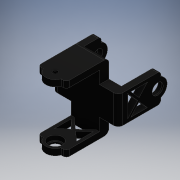
# Autodesk Inventor part: ServoArm
Saved by Autodesk Inventor 2016 (Build 200138000, 138)
## iProperties
Created: 2016-06-29
Part Number: ServoArm
Material: 一般
Document SubType Name: Modeling
Designer: Daisuke
Density: 1 g/cm^3
Appearance: 光沢 - 黒
Author: Daisuke
Autodesk Inventor part; units mm, degrees
ref_plane "YZ Plane" through (0, 0, 0) normal (1, 0, 0) x (0, 1, 0)
ref_plane "XZ Plane" through (0, 0, 0) normal (0, 1, 0) x (-1, 0, 0)
ref_plane "XY Plane" through (0, 0, 0) normal (0, 0, 1) x (1, 0, 0)
sketch "スケッチ1" plane through (0, 0, 0) normal (0, 1, 0) x (-1, 0, 0)
  line L0 (9, 20.9) -> (-9, 20.9)
  line L1 (-9, -20.9) -> (9, -20.9)
  line L2 (9, 20.9) -> (-9, -20.9) construction
  line L3 (-9, 20.9) -> (9, -20.9) construction
  line L4 (-20.9, 9) -> (-20.9, -9)
  line L5 (20.9, -9) -> (20.9, 9)
  line L6 (20.9, 9) -> (-20.9, -9) construction
  line L7 (-20.9, 9) -> (20.9, -9) construction
  line L8 (20.9, 9) -> (9, 9)
  line L9 (-9, 9) -> (-20.9, 9)
  line L10 (9, 9) -> (9, 20.9)
  line L11 (-9, 20.9) -> (-9, 9)
  line L12 (-9, -9) -> (-9, -20.9)
  line L13 (-20.9, -9) -> (-9, -9)
  line L14 (9, -9) -> (20.9, -9)
  line L15 (9, -20.9) -> (9, -9)
  point P0 (0, 0)
  dimension "d0" = 18
  dimension "d1" = 41.8
  dimension "d2" = 41.8
  dimension "d3" = 18
  constraints: 32 end point, 10 parallel, 4 midpoint, 4 perpendicular, 3 horizontal
  measures "d0" distance of L1.end L1.start
  measures "d1" distance of L1.start L0.end
  measures "d2" distance of L5.start L4.end
  measures "d3" distance of L4.end L4.start
extrude "押し出し1" add sketch "スケッチ1" along normal blind 6
sketch "スケッチ2" plane through (0, 6, 0) normal (0, 1, 0) x (1, 0, 0)
  line L0 (-20.9, -9) -> (-9, -9) projected
  line L1 (-9, 9) -> (-20.9, 9) projected
  line L2 (-20.9, -9) -> (-16.9, -9)
  line L3 (-16.9, -9) -> (-16.9, 9)
  line L4 (-16.9, 9) -> (-20.9, 9)
  line L5 (-20.9, 9) -> (-20.9, -9)
  line L6 (20.9, -9) -> (20.9, 9) projected
  line L7 (20.9, 9) -> (9, 9) projected
  line L8 (20.9, -9) -> (16.9, -9)
  line L9 (16.9, -9) -> (16.9, 9)
  line L10 (16.9, 9) -> (20.9, 9)
  line L11 (20.9, 9) -> (20.9, -9)
  point P0 (0, 0)
  dimension "d6" = 4
  dimension "d7" = 4
  constraints: 16 end point, 4 parallel, 2 horizontal, 2 perpendicular, 2 point on line
  measures "d6" distance of L4.end L3.end
  measures "d7" distance of L9.end L10.end
extrude "押し出し2" add sketch "スケッチ2" along normal blind 25
sketch "スケッチ3" plane through (0, 0, 0) normal (0, -1, 0) x (1, 0, 0)
  line L0 (-9, 20.9) -> (9, 20.9) projected
  line L1 (-9, 9) -> (-9, 20.9) projected
  line L2 (9, 20.9) -> (-9, 20.9)
  line L3 (-9, 20.9) -> (-9, 16.9)
  line L4 (-9, 16.9) -> (9, 16.9)
  line L5 (9, 16.9) -> (9, 20.9)
  line L6 (9, -9) -> (9, -20.9) projected
  line L7 (-9, -20.9) -> (-9, -9) projected
  line L8 (9, -20.9) -> (-9, -20.9)
  line L9 (-9, -20.9) -> (-9, -16.9)
  line L10 (-9, -16.9) -> (9, -16.9)
  line L11 (9, -16.9) -> (9, -20.9)
  point P0 (0, 0)
  dimension "d10" = 4
  dimension "d11" = 4
  constraints: 16 end point, 4 parallel, 2 horizontal, 2 perpendicular, 2 point on line
  measures "d10" distance of L3.end L2.end
  measures "d11" distance of L8.end L9.end
extrude "押し出し3" add sketch "スケッチ3" along normal blind 25
sketch "スケッチ4" plane through (20.9, 0, 9) normal (1, 0, 0) x (0, 0, -1)
  line L0 (9, 0) -> (9, 25) construction
  line L1 (9, 25) -> (15, 25) construction
  line L2 (9, 25) -> (0, 25) construction
  line L3 (0, 6) -> (0, 31) construction
  line L4 (0, 25) -> (2, 25) construction
  line L5 (9, 25) -> (18, 25) construction
  line L6 (18, 0) -> (18, 31) construction
  line L7 (18, 25) -> (16, 25) construction
  line L8 (2, 25) -> (0, 25) construction
  line L9 (18, 31) -> (0, 31) construction
  line L10 (9, 25) -> (9, 31) construction
  line L11 (0, 31) -> (18, 31) construction
  line L12 (0, 6) -> (0, 31) construction
  line L13 (0, 25) -> (0, 31) construction
  line L14 (18, 31) -> (0, 31) construction
  line L15 (0, 31) -> (18, 31) construction
  line L16 (18, 31) -> (18, 25) construction
  line L17 (0, 0) -> (0, 31) projected
  line L18 (0, 25) -> (0, 31)
  line L19 (0, 31) -> (18, 31)
  line L20 (18, 25) -> (18, 31)
  circle A0 centre (9, 25) radius 6
  line L21 (2, 27) -> (0, 27)
  line L22 (16, 27) -> (18, 27)
  line L23 (18, 6) -> (18, 31) projected
  line L24 (2, 27) -> (3.3431, 27)
  line L25 (14.6569, 27) -> (16, 27)
  circle A1 centre (9, 25) radius 1.5
  circle A2 centre (9, 25) radius 3
  dimension "d14" = 25
  dimension "d20" = 2
  dimension "d21" = 2
  dimension "d22" = 6
  dimension "d24" = 12
  dimension "d35" = 3
  dimension "d36" = 6
  constraints: 36 end point, 7 point on line, 5 coincident, 3 centre point, 3 collinear, 3 horizontal, 3 perpendicular, 2 point on circle, 2 vertical, 1 midpoint, 1 parallel
  measures "d14" distance of L0.start L0.end
  measures "d20" distance of L5.end L7.end
  measures "d21" distance of L8.start L2.end
  measures "d22" distance of L5.start L10.end
  measures "d24" diameter of A0
  measures "d35" diameter of A1
  measures "d36" diameter of A2
extrude "押し出し4" cut sketch "スケッチ4" against normal blind 41.8 contours L17 L19 A0 L24 L21 | L19 L20 L22 L25 A0
sketch "スケッチ5" plane through (-9, 6, 20.9) normal (0, 0, 1) x (1, 0, 0)
  line L0 (18, -31) -> (18, 0) projected
  line L1 (0, 0) -> (18, 0) projected
  line L2 (18, 0) -> (0, 0)
  line L3 (9, 0) -> (9, -25) construction
  line L4 (9, -25) -> (15, -25) construction
  line L5 (9, -25) -> (0, -25) construction
  line L6 (0, -6) -> (0, -31) construction
  line L7 (0, -25) -> (2, -25) construction
  line L8 (9, -25) -> (18, -25) construction
  line L9 (18, 0) -> (18, -31) construction
  line L10 (18, -25) -> (16, -25) construction
  line L11 (2, -25) -> (0, -25) construction
  line L12 (18, -31) -> (0, -31) construction
  line L13 (9, -25) -> (9, -31) construction
  line L14 (0, -31) -> (18, -31) construction
  line L15 (0, -6) -> (0, -31) construction
  line L16 (0, -25) -> (0, -31) construction
  line L17 (18, -31) -> (0, -31) construction
  line L18 (0, -31) -> (18, -31) construction
  line L19 (18, -31) -> (18, -25) construction
  line L20 (0, 0) -> (0, -31)
  line L21 (0, -25) -> (0, -31)
  line L22 (0, -31) -> (18, -31)
  line L23 (18, -25) -> (18, -31)
  circle A0 centre (9, -25) radius 6
  line L24 (2, -27) -> (0, -27)
  line L25 (16, -27) -> (18, -27)
  line L26 (18, -6) -> (18, -31)
  line L27 (2, -27) -> (3.3431, -27)
  line L28 (14.6569, -27) -> (16, -27)
  point P0 (9, -6)
  constraints: 54 end point, 7 point on line, 3 coincident, 2 point on circle, 1 centre point, 1 collinear
extrude "押し出し5" cut sketch "スケッチ5" against normal blind 41.8 contours L22 A0 L28 L25 L0 | L22 L20 L24 L27 A0
sketch "スケッチ6" plane through (-16.9, 6, 9) normal (1, 0, 0) x (0, 0, -1)
  line L0 (9, -0.0039) -> (9, 18.9961) construction
  line L1 (9, 18.9961) -> (15, 18.9961) construction
  line L2 (9, 18.9961) -> (0, 18.9961) construction
  line L3 (0, -0.0039) -> (0, 24.9961) construction
  line L4 (0, 18.9961) -> (2, 18.9961) construction
  line L5 (9, 18.9961) -> (18, 18.9961) construction
  line L6 (18, 18.9961) -> (18, 24.9961) construction
  line L7 (18, 18.9961) -> (16, 18.9961) construction
  line L8 (2, 18.9961) -> (0, 18.9961) construction
  line L9 (18, 24.9961) -> (0, 24.9961) construction
  line L10 (9, 18.9961) -> (9, 24.9961) construction
  line L11 (0, 24.9961) -> (18, 24.9961) construction
  line L12 (0, -0.0039) -> (0, 24.9961) construction
  line L13 (0, 18.9961) -> (0, 24.9961) construction
  line L14 (18, 24.9961) -> (0, 24.9961) construction
  line L15 (0, 24.9961) -> (18, 24.9961) construction
  line L16 (18, 24.9961) -> (18, 18.9961) construction
  line L17 (0, 18.9961) -> (0, 24.9961)
  line L18 (0, 18.9961) -> (0, 24.9961)
  line L19 (0, 24.9961) -> (18, 24.9961)
  line L20 (18, 18.9961) -> (18, 24.9961)
  circle A0 centre (9, 18.9961) radius 6
  line L21 (2, 20.9961) -> (0, 20.9961)
  line L22 (16, 20.9961) -> (18, 20.9961)
  line L23 (18, -0.0039) -> (18, 24.9961)
  line L24 (2, 20.9961) -> (3.3431, 20.9961)
  line L25 (14.6569, 20.9961) -> (16, 20.9961)
  circle A1 centre (9, 18.9961) radius 1.5
  circle A2 centre (9, 18.9961) radius 3
  point P0 (9, -6)
  dimension "d37" = 19
  dimension "d38" = 2
  dimension "d39" = 2
  dimension "d40" = 6
  dimension "d41" = 12
  dimension "d42" = 3
  dimension "d43" = 6
  constraints: 52 end point, 6 point on line, 5 coincident, 3 centre point, 3 collinear, 3 horizontal, 3 perpendicular, 2 point on circle, 2 vertical, 1 midpoint, 1 parallel
  measures "d37" distance of L0.start L0.end
  measures "d38" distance of L5.end L7.end
  measures "d39" distance of L2.end L8.start
  measures "d40" distance of L5.start L10.end
  measures "d41" diameter of A0
  measures "d42" diameter of A1
  measures "d43" diameter of A2
extrude "押し出し6" cut sketch "スケッチ6" against normal blind 4 and the other way blind 4 contours A1
sketch "スケッチ7" plane through (-16.9, 6, 9) normal (1, 0, 0) x (0, 0, -1)
  line L0 (9, -0.0039) -> (9, 18.9961) construction
  line L1 (9, 18.9961) -> (15, 18.9961) construction
  line L2 (9, 18.9961) -> (0, 18.9961) construction
  line L3 (0, -0.0039) -> (0, 24.9961) construction
  line L4 (0, 18.9961) -> (2, 18.9961) construction
  line L5 (9, 18.9961) -> (18, 18.9961) construction
  line L6 (18, 18.9961) -> (18, 24.9961) construction
  line L7 (18, 18.9961) -> (16, 18.9961) construction
  line L8 (2, 18.9961) -> (0, 18.9961) construction
  line L9 (18, 24.9961) -> (0, 24.9961) construction
  line L10 (9, 18.9961) -> (9, 24.9961) construction
  line L11 (0, 24.9961) -> (18, 24.9961) construction
  line L12 (0, -0.0039) -> (0, 24.9961) construction
  line L13 (0, 18.9961) -> (0, 24.9961) construction
  line L14 (18, 24.9961) -> (0, 24.9961) construction
  line L15 (0, 24.9961) -> (18, 24.9961) construction
  line L16 (18, 24.9961) -> (18, 18.9961) construction
  line L17 (0, 18.9961) -> (0, 24.9961)
  line L18 (0, 18.9961) -> (0, 24.9961)
  line L19 (0, 24.9961) -> (18, 24.9961)
  line L20 (18, 18.9961) -> (18, 24.9961)
  circle A0 centre (9, 18.9961) radius 6
  line L21 (2, 20.9961) -> (0, 20.9961)
  line L22 (16, 20.9961) -> (18, 20.9961)
  line L23 (18, -0.0039) -> (18, 24.9961)
  line L24 (2, 20.9961) -> (3.3431, 20.9961)
  line L25 (14.6569, 20.9961) -> (16, 20.9961)
  circle A1 centre (9, 18.9961) radius 1.5
  circle A2 centre (9, 18.9961) radius 3
  point P0 (9, -6)
  point P1 (9, -6)
  dimension "d48" = 19
  dimension "d49" = 2
  dimension "d50" = 2
  dimension "d51" = 6
  dimension "d52" = 12
  dimension "d53" = 3
  dimension "d54" = 6
  constraints: 52 end point, 6 point on line, 5 coincident, 3 centre point, 3 collinear, 3 horizontal, 3 perpendicular, 2 point on circle, 2 vertical, 1 midpoint, 1 parallel
  measures "d48" distance of L0.start L0.end
  measures "d49" distance of L5.end L7.end
  measures "d50" distance of L2.end L8.start
  measures "d51" distance of L5.start L10.end
  measures "d52" diameter of A0
  measures "d53" diameter of A1
  measures "d54" diameter of A2
extrude "押し出し7" cut sketch "スケッチ7" against normal blind 3 and the other way blind 3 contours A2
sketch "スケッチ8" plane through (9, 0, 16.9) normal (0, 0, -1) x (-1, 0, 0)
  line L0 (18, -25.0086) -> (18, -19.0086)
  line L1 (18, -25.0086) -> (18, -19.0086) construction
  line L2 (18, -19.0086) -> (18, -25.0086)
  line L3 (9, -19.0086) -> (15, -19.0086) construction
  line L4 (9, -19.0086) -> (18, -19.0086) construction
  line L5 (16, -21.0086) -> (18, -21.0086)
  line L6 (14.6569, -21.0086) -> (16, -21.0086)
  line L7 (9, -19.0086) -> (9, -25.0086) construction
  line L8 (2, -21.0086) -> (3.3431, -21.0086)
  line L9 (9, -19.0086) -> (0, -19.0086) construction
  line L10 (0, -19.0086) -> (0, -25.0086) construction
  line L11 (0, -19.0086) -> (0, -25.0086)
  circle A0 centre (9, -19.0086) radius 6
  line L12 (18, -19.0086) -> (18, -25.0086)
  line L13 (0, -19.0086) -> (0, -25.0086) construction
  line L14 (18, -19.0086) -> (18, -25.0086) construction
  line L15 (9, 0) -> (9, -25) construction
  line L16 (0, -19.0086) -> (0, -25.0086)
  line L17 (0, -0.0086) -> (0, -25.0086) construction
  line L18 (18, -25.0086) -> (0, -25.0086) construction
  line L19 (0, -25.0086) -> (18, -25.0086) construction
  line L20 (0, -25.0086) -> (18, -25.0086)
  line L21 (18, -25.0086) -> (0, -25.0086) construction
  line L22 (0, -25.0086) -> (18, -25.0086) construction
  line L23 (0, -19.0086) -> (2, -19.0086) construction
  line L24 (2, -19.0086) -> (0, -19.0086) construction
  line L25 (18, -19.0086) -> (16, -19.0086) construction
  line L26 (2, -21.0086) -> (0, -21.0086)
  circle A1 centre (9, -19.0086) radius 1.5
  circle A2 centre (9, -19.0086) radius 3
  point P0 (9, -0.0086)
  dimension "d59" = 3
  dimension "d60" = 6
  constraints: 54 end point, 6 point on line, 5 coincident, 3 centre point, 2 point on circle
  measures "d59" diameter of A1
  measures "d60" diameter of A2
extrude "押し出し8" cut sketch "スケッチ8" against normal blind 3 and the other way blind 3 contours A2
sketch "スケッチ9" plane through (9, 0, 16.9) normal (0, 0, -1) x (-1, 0, 0)
  line L0 (18, -25.0086) -> (18, -19.0086)
  line L1 (18, -25.0086) -> (18, -19.0086) construction
  line L2 (18, -19.0086) -> (18, -25.0086)
  line L3 (9, -19.0086) -> (15, -19.0086) construction
  line L4 (9, -19.0086) -> (18, -19.0086) construction
  line L5 (16, -21.0086) -> (18, -21.0086)
  line L6 (14.6569, -21.0086) -> (16, -21.0086)
  line L7 (9, -19.0086) -> (9, -25.0086) construction
  line L8 (2, -21.0086) -> (3.3431, -21.0086)
  line L9 (9, -19.0086) -> (0, -19.0086) construction
  line L10 (0, -19.0086) -> (0, -25.0086) construction
  line L11 (0, -19.0086) -> (0, -25.0086)
  circle A0 centre (9, -19.0086) radius 6
  line L12 (18, -19.0086) -> (18, -25.0086)
  line L13 (0, -19.0086) -> (0, -25.0086) construction
  line L14 (18, -19.0086) -> (18, -25.0086) construction
  line L15 (9, 0) -> (9, -25) construction
  line L16 (0, -19.0086) -> (0, -25.0086)
  line L17 (0, -0.0086) -> (0, -25.0086) construction
  line L18 (18, -25.0086) -> (0, -25.0086) construction
  line L19 (0, -25.0086) -> (18, -25.0086) construction
  line L20 (0, -25.0086) -> (18, -25.0086)
  line L21 (18, -25.0086) -> (0, -25.0086) construction
  line L22 (0, -25.0086) -> (18, -25.0086) construction
  line L23 (0, -19.0086) -> (2, -19.0086) construction
  line L24 (2, -19.0086) -> (0, -19.0086) construction
  line L25 (18, -19.0086) -> (16, -19.0086) construction
  line L26 (2, -21.0086) -> (0, -21.0086)
  circle A1 centre (9, -19.0086) radius 1.5
  circle A2 centre (9, -19.0086) radius 3
  point P0 (9, -0.0086)
  dimension "d65" = 3
  dimension "d66" = 6
  constraints: 54 end point, 6 point on line, 5 coincident, 3 centre point, 2 point on circle
  measures "d65" diameter of A1
  measures "d66" diameter of A2
extrude "押し出し9" cut sketch "スケッチ9" against normal blind 4 and the other way blind 37.8 contours A1
sketch "スケッチ10" plane through (-9, 0, -16.9) normal (0, 0, 1) x (1, 0, 0)
  line L0 (18, -25.0086) -> (18, -19.0086)
  line L1 (18, -25.0086) -> (18, -19.0086) construction
  line L2 (18, -19.0086) -> (18, -25.0086)
  line L3 (9, -19.0086) -> (15, -19.0086) construction
  line L4 (9, -19.0086) -> (18, -19.0086) construction
  line L5 (16, -21.0086) -> (18, -21.0086)
  line L6 (14.6569, -21.0086) -> (16, -21.0086)
  line L7 (9, -19.0086) -> (9, -25.0086) construction
  line L8 (2, -21.0086) -> (3.3431, -21.0086)
  line L9 (9, -19.0086) -> (0, -19.0086) construction
  line L10 (0, -19.0086) -> (0, -25.0086) construction
  line L11 (0, -19.0086) -> (0, -25.0086)
  circle A0 centre (9, -19.0086) radius 6
  line L12 (18, -19.0086) -> (18, -25.0086)
  line L13 (0, -19.0086) -> (0, -25.0086) construction
  line L14 (18, -19.0086) -> (18, -25.0086) construction
  line L15 (9, 0) -> (9, -25) construction
  line L16 (0, -19.0086) -> (0, -25.0086)
  line L17 (0, -0.0086) -> (0, -25.0086) construction
  line L18 (18, -25.0086) -> (0, -25.0086) construction
  line L19 (0, -25.0086) -> (18, -25.0086) construction
  line L20 (0, -25.0086) -> (18, -25.0086)
  line L21 (18, -25.0086) -> (0, -25.0086) construction
  line L22 (0, -25.0086) -> (18, -25.0086) construction
  line L23 (0, -19.0086) -> (2, -19.0086) construction
  line L24 (2, -19.0086) -> (0, -19.0086) construction
  line L25 (18, -19.0086) -> (16, -19.0086) construction
  line L26 (2, -21.0086) -> (0, -21.0086)
  circle A1 centre (9, -19.0086) radius 3.5
  circle A2 centre (9, -19.0086) radius 4.5
  point P0 (9, -0.0086)
  dimension "d71" = 7
  dimension "d72" = 9
  constraints: 54 end point, 6 point on line, 5 coincident, 3 centre point, 2 point on circle
  measures "d71" diameter of A1
  measures "d72" diameter of A2
extrude "押し出し10" cut sketch "スケッチ10" against normal blind 4 contours A1
sketch "スケッチ11" plane through (-9, 0, -16.9) normal (0, 0, 1) x (1, 0, 0)
  line L0 (18, -25.0086) -> (18, -19.0086)
  line L1 (18, -25.0086) -> (18, -19.0086) construction
  line L2 (18, -19.0086) -> (18, -25.0086)
  line L3 (9, -19.0086) -> (15, -19.0086) construction
  line L4 (9, -19.0086) -> (18, -19.0086) construction
  line L5 (16, -21.0086) -> (18, -21.0086)
  line L6 (14.6569, -21.0086) -> (16, -21.0086)
  line L7 (9, -19.0086) -> (9, -25.0086) construction
  line L8 (2, -21.0086) -> (3.3431, -21.0086)
  line L9 (9, -19.0086) -> (0, -19.0086) construction
  line L10 (0, -19.0086) -> (0, -25.0086) construction
  line L11 (0, -19.0086) -> (0, -25.0086)
  circle A0 centre (9, -19.0086) radius 6
  line L12 (18, -19.0086) -> (18, -25.0086)
  line L13 (0, -19.0086) -> (0, -25.0086) construction
  line L14 (18, -19.0086) -> (18, -25.0086) construction
  line L15 (9, 0) -> (9, -25) construction
  line L16 (0, -19.0086) -> (0, -25.0086)
  line L17 (0, -0.0086) -> (0, -25.0086) construction
  line L18 (18, -25.0086) -> (0, -25.0086) construction
  line L19 (0, -25.0086) -> (18, -25.0086) construction
  line L20 (0, -25.0086) -> (18, -25.0086)
  line L21 (18, -25.0086) -> (0, -25.0086) construction
  line L22 (0, -25.0086) -> (18, -25.0086) construction
  line L23 (0, -19.0086) -> (2, -19.0086) construction
  line L24 (2, -19.0086) -> (0, -19.0086) construction
  line L25 (18, -19.0086) -> (16, -19.0086) construction
  line L26 (2, -21.0086) -> (0, -21.0086)
  circle A1 centre (9, -19.0086) radius 3.5
  circle A2 centre (9, -19.0086) radius 4.5
  point P0 (9, -0.0086)
  dimension "d75" = 7
  dimension "d76" = 9
  constraints: 54 end point, 6 point on line, 5 coincident, 3 centre point, 2 point on circle
  measures "d75" diameter of A1
  measures "d76" diameter of A2
extrude "押し出し11" cut sketch "スケッチ11" against normal blind 3 contours A2
sketch "スケッチ12" plane through (-9, 0, -16.9) normal (0, 0, 1) x (1, 0, 0)
  line L0 (18, -25.0086) -> (18, -19.0086)
  line L1 (18, -25.0086) -> (18, -19.0086) construction
  line L2 (18, -19.0086) -> (18, -25.0086)
  line L3 (9, -19.0086) -> (15, -19.0086) construction
  line L4 (9, -19.0086) -> (18, -19.0086) construction
  line L5 (16, -21.0086) -> (18, -21.0086)
  line L6 (14.6569, -21.0086) -> (16, -21.0086)
  line L7 (9, -19.0086) -> (9, -25.0086) construction
  line L8 (2, -21.0086) -> (3.3431, -21.0086)
  line L9 (9, -19.0086) -> (0, -19.0086) construction
  line L10 (0, -19.0086) -> (0, -25.0086) construction
  line L11 (0, -19.0086) -> (0, -25.0086)
  circle A0 centre (9, -19.0086) radius 6
  line L12 (18, -19.0086) -> (18, -25.0086)
  line L13 (0, -19.0086) -> (0, -25.0086) construction
  line L14 (18, -19.0086) -> (18, -25.0086) construction
  line L15 (9, 0) -> (9, -25) construction
  line L16 (0, -19.0086) -> (0, -25.0086)
  line L17 (0, -0.0086) -> (0, -25.0086) construction
  line L18 (18, -25.0086) -> (0, -25.0086) construction
  line L19 (0, -25.0086) -> (18, -25.0086) construction
  line L20 (0, -25.0086) -> (18, -25.0086)
  line L21 (18, -25.0086) -> (0, -25.0086) construction
  line L22 (0, -25.0086) -> (18, -25.0086) construction
  line L23 (0, -19.0086) -> (2, -19.0086) construction
  line L24 (2, -19.0086) -> (0, -19.0086) construction
  line L25 (18, -19.0086) -> (16, -19.0086) construction
  line L26 (2, -21.0086) -> (0, -21.0086)
  circle A1 centre (9, -19.0086) radius 3.5
  circle A2 centre (9, -19.0086) radius 4.5
  line L27 (18, -19.0086) -> (16, -19.0086) construction
  line L28 (0, 0) -> (18, 0) construction
  line L29 (18, 0) -> (18, -21) construction
  line L30 (0, 0) -> (18, 0) construction
  line L31 (18, 0) -> (18, -14.5086) construction
  line L32 (0, -14.5086) -> (0, 0) construction
  line L33 (18, 0) -> (16, 0) construction
  line L34 (0, 0) -> (2, 0) construction
  line L35 (16, 0) -> (2, 0)
  line L36 (2, -2) -> (2, -12.5086)
  line L37 (16, -12.5086) -> (16, -2)
  line L38 (16, -12.5086) -> (10.1192, -7.2543)
  line L39 (9, -6.2543) -> (2, 0)
  line L40 (16, -2) -> (10.1192, -7.2543)
  line L41 (9, -8.2543) -> (2, -14.5086)
  line L42 (2, -12.5086) -> (7.8808, -7.2543)
  line L43 (9, -6.2543) -> (16, 0)
  line L44 (2, -2) -> (7.8808, -7.2543)
  line L45 (9, -8.2543) -> (16, -14.5086)
  line L46 (2, -14.5086) -> (9, -14.5086)
  line L47 (12.9686, -14.5086) -> (16, -14.5086)
  line L48 (18, -14.5086) -> (9, -14.5086) construction
  line L49 (5.0314, -14.5086) -> (0, -14.5086) construction
  point P0 (9, -0.0086)
  dimension "d80" = 9
  dimension "d79" = 7
  dimension "d81" = 2
  dimension "d83" = 2
  constraints: 96 end point, 14 parallel, 12 point on line, 5 coincident, 4 point on circle, 2 centre point, 2 horizontal, 2 perpendicular, 1 collinear, 1 vertical alignment, 2 other
  measures "d79" diameter of A1
  measures "d81" distance of L0.end L25.end
  measures "d83" distance of L28.start L34.end
extrude "押し出し12" cut sketch "スケッチ12" against normal blind 4 contours L43 L39 L35 | L44 L42 L36 | L38 L40 L37
sketch "スケッチ13" plane through (16.9, 6, -9) normal (-1, 0, 0) x (0, 0, 1)
  line L0 (0, 0) -> (18, 0) construction
  line L1 (0, 0) -> (18, 0) construction
  line L2 (18, 0) -> (16, 0) construction
  line L3 (0, 0) -> (2, 0) construction
  line L4 (16, 0) -> (2, 0)
  line L5 (18, 25.0086) -> (18, 19.0086)
  line L6 (18, 25.0086) -> (18, 19.0086) construction
  line L7 (18, 19.0086) -> (18, 25.0086)
  line L8 (9, 19.0086) -> (15, 19.0086) construction
  line L9 (9, 19.0086) -> (18, 19.0086) construction
  line L10 (16, 21.0086) -> (18, 21.0086)
  line L11 (14.6569, 21.0086) -> (16, 21.0086)
  line L12 (9, 19.0086) -> (9, 25.0086) construction
  line L13 (2, 21.0086) -> (3.3431, 21.0086)
  line L14 (9, 19.0086) -> (0, 19.0086) construction
  line L15 (0, 19.0086) -> (0, 25.0086) construction
  line L16 (0, 19.0086) -> (0, 25.0086)
  circle A0 centre (9, 19.0086) radius 6
  line L17 (18, 19.0086) -> (18, 25.0086)
  line L18 (0, 19.0086) -> (0, 25.0086) construction
  line L19 (18, 19.0086) -> (18, 25.0086) construction
  line L20 (9, 0) -> (9, 25) construction
  line L21 (0, 19.0086) -> (0, 25.0086)
  line L22 (0, 0.0086) -> (0, 25.0086) construction
  line L23 (18, 25.0086) -> (0, 25.0086) construction
  line L24 (0, 25.0086) -> (18, 25.0086) construction
  line L25 (0, 25.0086) -> (18, 25.0086)
  line L26 (18, 25.0086) -> (0, 25.0086) construction
  line L27 (0, 25.0086) -> (18, 25.0086) construction
  line L28 (0, 19.0086) -> (2, 19.0086) construction
  line L29 (2, 19.0086) -> (0, 19.0086) construction
  line L30 (18, 19.0086) -> (16, 19.0086) construction
  line L31 (2, 21.0086) -> (0, 21.0086)
  circle A1 centre (9, 19.0086) radius 3.5
  circle A2 centre (9, 19.0086) radius 4.5
  line L32 (18, 19.0086) -> (16, 19.0086) construction
  line L33 (18, 0) -> (18, 21) construction
  line L34 (18, 0) -> (18, 14.5086) construction
  line L35 (0, 14.5086) -> (0, 0) construction
  line L36 (2, 2) -> (2, 12.5086)
  line L37 (16, 12.5086) -> (16, 2)
  line L38 (16, 12.5086) -> (10.1192, 7.2543)
  line L39 (9, 6.2543) -> (2, 0)
  line L40 (16, 2) -> (10.1192, 7.2543)
  line L41 (9, 8.2543) -> (2, 14.5086)
  line L42 (2, 12.5086) -> (7.8808, 7.2543)
  line L43 (9, 6.2543) -> (16, 0)
  line L44 (2, 2) -> (7.8808, 7.2543)
  line L45 (9, 8.2543) -> (16, 14.5086)
  line L46 (2, 14.5086) -> (9, 14.5086)
  line L47 (12.9686, 14.5086) -> (16, 14.5086)
  line L48 (18, 14.5086) -> (9, 14.5086) construction
  line L49 (5.0314, 14.5086) -> (0, 14.5086) construction
  line L50 (18, 0) -> (18, -1.7869) construction
  line L51 (18, 0) -> (18, -1.7869) construction
  line L52 (18, -14.2956) -> (18, -14.5086) construction
  point P0 (9, -0.0086)
  point P1 (9, -25)
  point P2 (9, 6)
  point P3 (9, 0.0086)
  dimension "d93" = 2
  constraints: 106 end point, 13 point on line, 5 coincident, 4 point on circle, 3 symmetric about line, 2 centre point, 2 horizontal, 2 perpendicular, 1 vertical alignment, 2 other
  measures "d93" distance of L0.start L3.end
extrude "押し出し13" cut sketch "スケッチ13" against normal blind 4 contours L4 L39 L43 | A1 | L36 L42 L44 | L37 L40 L38
sketch "スケッチ14" plane through (16.9, 6, 9) normal (-1, 0, 0) x (0, 0, 1)
  line L0 (18, -14.2956) -> (18, -14.5086) construction
  line L1 (0, 0) -> (-18, 0) construction
  line L2 (0, 0) -> (-18, 0) construction
  line L3 (-18, 0) -> (-16, 0) construction
  line L4 (0, 0) -> (-2, 0) construction
  line L5 (-16, 0) -> (-2, 0)
  line L6 (-18, 25.0086) -> (-18, 19.0086)
  line L7 (-14.6569, 21.0086) -> (-16, 21.0086)
  line L8 (-18, 25.0086) -> (-18, 19.0086) construction
  line L9 (-18, 19.0086) -> (-18, 25.0086)
  line L10 (-16, 21.0086) -> (-18, 21.0086)
  line L11 (-9, 19.0086) -> (-15, 19.0086) construction
  line L12 (-9, 19.0086) -> (-18, 19.0086) construction
  line L13 (-9, 19.0086) -> (-9, 25.0086) construction
  line L14 (0, 25.0086) -> (-18, 25.0086) construction
  line L15 (-18, 25.0086) -> (0, 25.0086) construction
  line L16 (0, 25.0086) -> (-18, 25.0086) construction
  line L17 (0, 25.0086) -> (-18, 25.0086)
  line L18 (-18, 25.0086) -> (0, 25.0086) construction
  circle A0 centre (-9, 19.0086) radius 3.5
  circle A1 centre (-9, 19.0086) radius 4.5
  line L19 (-9, 19.0086) -> (0, 19.0086) construction
  line L20 (-2, 21.0086) -> (-3.3431, 21.0086)
  line L21 (-2, 21.0086) -> (0, 21.0086)
  line L22 (-18, 19.0086) -> (-18, 25.0086) construction
  line L23 (-18, 19.0086) -> (-18, 25.0086)
  line L24 (-2, 19.0086) -> (0, 19.0086) construction
  line L25 (0, 19.0086) -> (-2, 19.0086) construction
  line L26 (-9, 6.2543) -> (-16, 0)
  line L27 (-16, 2) -> (-10.1192, 7.2543)
  line L28 (-16, 12.5086) -> (-10.1192, 7.2543)
  line L29 (-16, 12.5086) -> (-16, 2)
  line L30 (-12.9686, 14.5086) -> (-16, 14.5086)
  line L31 (-9, 8.2543) -> (-16, 14.5086)
  line L32 (-18, 14.5086) -> (-9, 14.5086) construction
  circle A2 centre (-9, 19.0086) radius 6
  line L33 (-9, 0) -> (-9, 25) construction
  line L34 (-18, 19.0086) -> (-16, 19.0086) construction
  line L35 (-18, 19.0086) -> (-16, 19.0086) construction
  line L36 (-18, 0) -> (-18, 21) construction
  line L37 (-18, 0) -> (-18, 14.5086) construction
  line L38 (-9, 6.2543) -> (-2, 0)
  line L39 (-2, 12.5086) -> (-7.8808, 7.2543)
  line L40 (-2, 2) -> (-2, 12.5086)
  line L41 (-2, 14.5086) -> (-9, 14.5086)
  line L42 (-9, 8.2543) -> (-2, 14.5086)
  line L43 (-2, 2) -> (-7.8808, 7.2543)
  line L44 (-5.0314, 14.5086) -> (0, 14.5086) construction
  line L45 (-18, 0) -> (-18, -1.7869) construction
  line L46 (-18, 0) -> (-18, -1.7869) construction
  point P0 (-9, -6)
  point P1 (9, -25)
  point P2 (-9, -0.0086)
  point P3 (-9, 6)
  point P4 (-9, 0.0086)
  constraints: 94 end point, 11 point on line, 5 coincident, 4 point on circle, 2 centre point, 1 vertical alignment, 2 other
extrude "押し出し14" cut sketch "スケッチ14" against normal blind 3 contours A1
fillet "フィレット1" radius 2 6 edges at (-9, -21, 18.9) (9, -21, 18.9) (-9, -21, -18.9) (9, -21, -18.9) (18.9, 27, 9) (-18.9, 27, 9)
fillet "フィレット2" radius 3 4 edges at (0, 6, 20.9) (0, 6, -20.9) (20.9, 0, 0) (-20.9, 0, 0)
